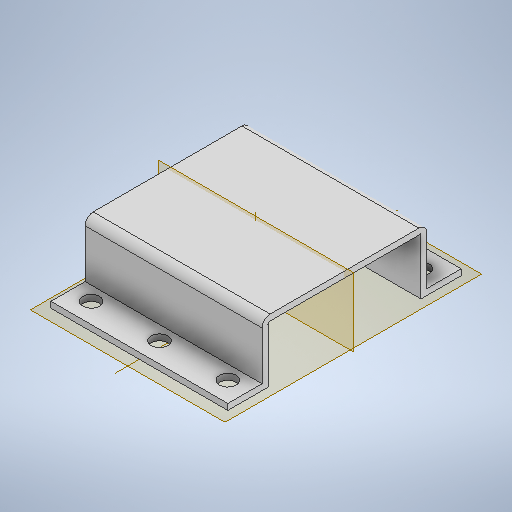
# Autodesk Inventor part: connector-houseing-top-cover
Saved by Autodesk Inventor 2025 (Build 290162000, 162)
## iProperties
Created: 2025-05-30
Part Number: connector-houseing-top-cover
Material: Generic
Document SubType Name: Modeling
Designer: mumin
Density: 1 g/cm^3
Appearance: Default
Author: mumin
Autodesk Inventor part; units mm, degrees
ref_plane "YZ Plane" through (0, 0, 0) normal (1, 0, 0) x (0, 1, 0)
sketch "Sketch2" plane through (0, 0, 0) normal (1, 0, 0) x (0, 1, 0)
  line L0 (0, 19) -> (0, 29)
  line L1 (0, 29) -> (1.5, 29)
  line L2 (1.5, 29) -> (1.5, 20.5)
  line L3 (0, 19) -> (13.5, 19)
  line L4 (14, 18.5) -> (14, 0)
  line L5 (1.5, 20.5) -> (13.5, 20.5)
  line L6 (15.5, 18.5) -> (15.5, 0)
  line L7 (-3.1828, 0) -> (19.0971, 0) projected
  line L8 (0, -40.6) -> (0, 40.6) projected
  line L9 (0, -19) -> (0, -29)
  line L10 (0, -29) -> (1.5, -29)
  line L11 (1.5, -29) -> (1.5, -20.5)
  line L12 (0, -19) -> (14, -19)
  line L13 (14, -19) -> (14, 0)
  line L14 (1.5, -20.5) -> (13.5, -20.5)
  line L15 (15.5, -18.5) -> (15.5, 0)
  arc A0 (15.5, 18.5) -> (13.5, 20.5) centre (13.5, 18.5) ccw
  arc A1 (13.5, -20.5) -> (15.5, -18.5) centre (13.5, -18.5) ccw
  arc A2 (14, 18.5) -> (13.5, 19) centre (13.5, 18.5) ccw
  point P0 (0, 0)
  point P1 (14, 19)
  point P2 (15.5, 20.5)
  point P3 (15.5, -20.5)
  point P4 (0, 26.5)
  point P5 (2.5, -19)
  point P6 (0, 19)
  dimension "d0" = 10
  dimension "d1" = 1.5
  dimension "d2" = 8.5
  dimension "d4" = 14
  dimension "d5" = 19
  dimension "d6" = 1.5
  dimension "d7" = 2
  dimension "d22" = 0.5
  constraints: 28 end point, 10 point on line, 6 point on circle, 6 symmetric about line, 6 tangent, 4 perpendicular, 3 centre point, 2 horizontal, 1 collinear, 1 equal radius, 1 vertical
  measures "d0" distance of L0.start L0.end
  measures "d1" distance of L0.end L1.end
  measures "d2" distance of L2.end L1.end
  measures "d4" distance of L0.start point (14, 19)
  measures "d5" distance of point (14, 19) L4.end
  measures "d6" distance between parallel lines of L4 L6
  measures "d7" radius of A0
  measures "d22" radius of A2
extrude "Extrusion1" add sketch "Sketch2" along normal mid plane 44 contours L0 L1 L2 L5 A0 L6 L7 L4 A2 L3 | L7 L15 A1 L14 L11 L10 L8 L12 L13
sketch "Sketch3" plane through (-22, 0, 19) normal (0, -1, 0) x (1, 0, 0)
  line L0 (0, 10) -> (44, 10) projected
  line L1 (22, -59.6) -> (22, 21.6) projected
  point P0 (22, -19)
  point P1 (22, 5)
  point P2 (39, 5)
  point P3 (5, 5)
  dimension "d10" = 5
  dimension "d12" = 17
  dimension "d14" = 5
  dimension "d23" = 17
  dimension "d24" = 5
  measures "d10" distance from line of L0 point (22, 5)
  measures "d12" distance of point (39, 5) point (22, 5)
  measures "d14" distance from line of L0 point (39, 5)
  measures "d23" distance from line of point (5, 5) L1
  measures "d24" distance from line of L0 point (5, 5)
hole "Hole1" at (0, 0, 24) at (17, 0, 24) at (-17, 0, 24) direction (0, 1, 0) diameter 4.2 end through all
mirror "Mirror1" about plane through (0, 0, 0) normal (0, 0, 1) of "Hole1"
body "Solid1"
